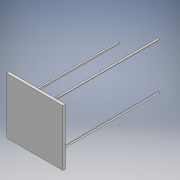
# Autodesk Inventor part: 底座
Saved by Autodesk Inventor 2017 (Build 210142000, 142)
## iProperties
Part Number: 底座
Material: 一般
Document SubType Name: Modeling
Designer: Brian
Density: 1 g/cm^3
Appearance: 預設
Author: Brian
Autodesk Inventor part; units mm, degrees
ref_plane "YZ Plane" through (0, 0, 0) normal (1, 0, 0) x (0, 1, 0)
ref_plane "XZ Plane" through (0, 0, 0) normal (0, 1, 0) x (-1, 0, 0)
ref_plane "XY Plane" through (0, 0, 0) normal (0, 0, 1) x (1, 0, 0)
sketch "草圖1" plane through (0, 0, 0) normal (0, 1, 0) x (-1, 0, 0)
  circle A0 centre (0, 0) radius 200
  dimension "d0" = 400
  constraints: 1 centre point, 1 coincident
  measures "d0" diameter of A0
extrude "擠出1" add sketch "草圖1" along normal blind 5
sketch "草圖2" plane through (0, 5, 0) normal (0, 1, 0) x (1, 0, 0)
  line L0 (-205, 5) -> (-195, 5)
  line L1 (-195, 5) -> (-195, -5)
  line L2 (-195, -5) -> (-205, -5)
  line L3 (-205, -5) -> (-205, 5)
  circle A0 centre (0, 0) radius 200 projected
  line L4 (-205, 5) -> (-195, -5) construction
  line L5 (-195, 5) -> (-205, -5) construction
  point P0 (-200, 0)
  dimension "d3" = 10
  dimension "d4" = 10
  constraints: 12 end point, 2 midpoint, 2 parallel, 1 horizontal, 1 horizontal alignment, 1 perpendicular, 1 other
  measures "d3" distance of L0.end L1.end
  measures "d4" distance of L0.start L0.end
extrude "擠出2" add sketch "草圖2" along normal blind 800 and the other way blind 5 contours L0 A0 L2 L3 | L0 L1 L2 A0 picked at (-196.6644, -0.5556)
pattern_circular "環形陣列1" count 3 over 360 about axis through (0, 0, 0) along (0, 1, 0) of "擠出2"
sketch "草圖3" plane through (0, 0, 0) normal (0, -1, 0) x (1, 0, 0)
  line L0 (-200, 200) -> (200, 200)
  line L1 (200, 200) -> (200, -200)
  line L2 (200, -200) -> (-200, -200)
  line L3 (-200, -200) -> (-200, 200)
  line L4 (-200, 200) -> (200, -200) construction
  line L5 (200, 200) -> (-200, -200) construction
  point P0 (0, 0)
  dimension "d12" = 400
  dimension "d13" = 400
  constraints: 12 end point, 2 midpoint, 2 parallel, 1 horizontal, 1 perpendicular
  measures "d12" distance of L0.end L1.end
  measures "d13" distance of L1.end L2.end
extrude "擠出3" add sketch "草圖3" along normal blind 20
sketch "草圖4" plane through (0, -20, 0) normal (0, -1, 0) x (1, 0, 0)
  line L0 (-210, 210) -> (210, 210)
  line L1 (210, 210) -> (210, -210)
  line L2 (210, -210) -> (-210, -210)
  line L3 (-210, -210) -> (-210, 210)
  line L4 (-210, 210) -> (210, -210) construction
  line L5 (210, 210) -> (-210, -210) construction
  point P0 (0, 0)
  dimension "d16" = 420
  dimension "d17" = 420
  constraints: 12 end point, 2 midpoint, 2 parallel, 1 horizontal, 1 perpendicular
  measures "d16" distance of L0.end L1.end
  measures "d17" distance of L1.end L2.end
extrude "擠出4" add sketch "草圖4" against normal up to surface (20 mm away)
